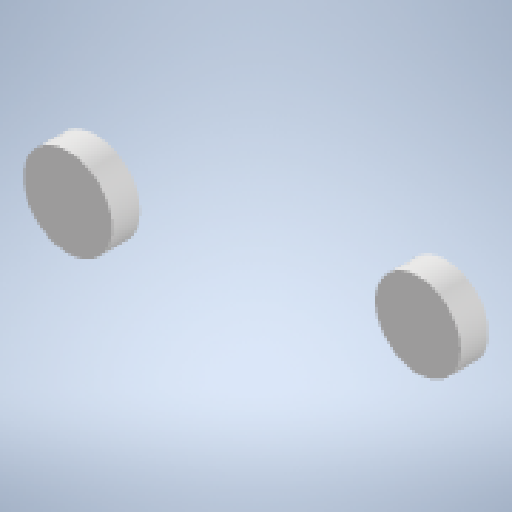
# Autodesk Inventor part: EyesGoma
Saved by Autodesk Inventor 2023 (Build 270158000, 158)
## iProperties
Created: 2022-11-10
Part Number: EyesGoma
Material: Generic
Document SubType Name: Modeling
Designer: reide
Density: 1 g/cm^3
Appearance: Default
Author: reide
Autodesk Inventor part; units mm, degrees
ref_plane "YZ Plane" through (0, 0, 0) normal (1, 0, 0) x (0, 1, 0)
ref_plane "XZ Plane" through (0, 0, 0) normal (0, 1, 0) x (-1, 0, 0)
ref_plane "XY Plane" through (0, 0, 0) normal (0, 0, 1) x (1, 0, 0)
sketch "Sketch1" plane through (0, 0, 0) normal (0, 0, 1) x (1, 0, 0)
  arc A0 (31.1669, -27.5722) -> (35.8875, -22.8773) centre (21.6106, -13.2427) ccw projected
  arc A1 (35.8875, -22.8773) -> (34.8455, -21.6033) centre (-10.0066, -59.351) ccw projected
  line L0 (31.177, -26.5722) -> (-3.0608, -26.5722) projected
  arc A2 (-3.0608, -26.5722) -> (-3.3209, -25.2629) centre (-5.1893, -26.3146) ccw projected
  arc A3 (-3.3209, -25.2629) -> (-1.1986, -22.6985) centre (-4.2539, -22.3302) ccw projected
  arc A4 (-1.1986, -22.6985) -> (27.6561, -16.2412) centre (3.0649, 25.9479) ccw projected
  arc A5 (34.8455, -21.6033) -> (38.4558, -17.1259) centre (14.65, -1.6245) ccw projected
  arc A6 (29.6868, -16.1644) -> (34.1879, -20.9364) centre (42.4009, -8.681) ccw projected
  arc A7 (29.6868, -16.1644) -> (32.1813, -14.508) centre (22.6557, -2.8691) ccw projected
  arc A8 (36.2837, -17.718) -> (32.1813, -14.508) centre (33.8318, -16.6251) ccw projected
  arc A9 (38.4558, -17.1259) -> (37.2045, -13.6874) centre (36.2505, -15.9815) ccw projected
  arc A10 (36.3385, -10.6874) -> (37.2045, -13.6874) centre (37.9725, -11.8408) ccw projected
  arc A11 (36.3385, -10.6874) -> (35.7081, 6.3323) centre (24.8683, -2.5908) ccw projected
  arc A12 (35.7081, 6.3323) -> (31.4684, 20.3428) centre (7.4536, 5.4291) ccw projected
  arc A13 (31.4684, 20.3428) -> (30.4027, 34.135) centre (0, 24.8485) ccw projected
  arc A14 (30.4027, 34.135) -> (17.0904, 32.0182) centre (26.8002, 13.8731) ccw projected
  arc A15 (17.0904, 32.0182) -> (-22.1361, 25.4066) centre (3.3472, -6.1143) ccw projected
  arc A16 (-22.1361, 25.4066) -> (-37.0956, 22.1531) centre (-24.1189, -1.495) ccw projected
  arc A17 (-37.0956, 22.1531) -> (-33.3027, 6.5823) centre (17.6972, 27.2528) ccw projected
  arc A18 (-33.3027, 6.5823) -> (-30.2964, -14.6197) centre (2.7199, 0.876) ccw projected
  arc A19 (-30.2964, -14.6197) -> (-18.2146, -23.7335) centre (-13.8358, -5.3636) ccw projected
  arc A20 (-18.2146, -23.7335) -> (-18.242, -27.5722) centre (-11.8923, -25.698) ccw projected
  line L1 (-44.3323, -27.5722) -> (-18.242, -27.5722) projected
  arc A21 (-44.3323, -27.5722) -> (-48.3323, -31.5722) centre (-44.3323, -31.5722) ccw projected
  line L2 (-48.3323, -136.5722) -> (-48.3323, -31.5722) projected
  arc A22 (-48.3323, -136.5722) -> (-44.3323, -140.5722) centre (-44.3323, -136.5722) ccw projected
  line L3 (92.8689, -140.5722) -> (-44.3323, -140.5722) projected
  line L4 (92.8689, -132.5706) -> (92.8689, -140.5722) projected
  line L5 (-38.9073, -132.5706) -> (92.8689, -132.5706) projected
  arc A23 (-40.9073, -130.5706) -> (-38.9073, -132.5706) centre (-38.9073, -130.5706) ccw projected
  line L6 (-40.9073, -37.5722) -> (-40.9073, -130.5706) projected
  arc A24 (-38.9073, -35.5722) -> (-40.9073, -37.5722) centre (-38.9073, -37.5722) ccw projected
  line L7 (92.8689, -35.5722) -> (-38.9073, -35.5722) projected
  line L8 (92.8689, -27.5722) -> (92.8689, -35.5722) projected
  line L9 (31.1669, -27.5722) -> (92.8689, -27.5722) projected
  arc A25 (10.4658, -0.0889) -> (9.3999, 0) centre (9.9366, 0) ccw projected
  arc A26 (10.4658, -0.0889) -> (10.6052, -0.4853) centre (11.0805, -0.0954) ccw projected
  arc A27 (10.6052, -0.4853) -> (12.2217, -0.0769) centre (11.2935, 0.1936) ccw projected
  arc A28 (14.0708, 0) -> (12.2217, -0.0769) centre (13.1642, -0.4715) ccw projected
  arc A29 (14.0708, 0) -> (15.5201, 0.876) centre (14.6273, 0.7161) ccw projected
  arc A30 (16.6059, 1.2358) -> (15.5201, 0.876) centre (16.0433, 1.1154) ccw projected
  arc A31 (13.0987, -0.702) -> (16.6059, 1.2358) centre (14.6781, 0.5822) ccw projected
  arc A32 (9.3999, 0) -> (13.0987, -0.702) centre (11.2957, -0.1065) ccw projected
  arc A33 (30.6396, 22.3597) -> (19.6168, 31.4004) centre (6.9952, 4.7714) ccw projected
  arc A34 (29.7697, 32.8548) -> (19.6168, 31.4004) centre (27.3183, 13.8041) ccw projected
  arc A35 (30.6396, 22.3597) -> (29.7697, 32.8548) centre (2.7, 25.3277) ccw projected
  line L10 (-7.4612, -26.5722) -> (-17.5392, -26.5722) projected
  arc A36 (-9.2038, -17.0917) -> (-15.8005, -20.192) centre (-6.8054, -30.7634) ccw projected
  arc A37 (-4.9865, -25.698) -> (-9.2038, -17.0917) centre (-21.6299, -28.5174) ccw projected
  arc A38 (-4.9865, -25.698) -> (-7.4612, -26.5722) centre (2.3833, -50.5016) ccw projected
  circle A39 centre (24.8683, 4.8774) radius 3.1762 projected
  circle A40 centre (0, 0) radius 3.3209 projected
  arc A41 (-23.3023, 23.7394) -> (-30.7067, 8.9093) centre (205.8131, -99.9189) ccw projected
  arc A42 (-35.2106, 21.0181) -> (-30.7067, 8.9093) centre (-10.6119, 23.2756) ccw projected
  arc A43 (-23.3023, 23.7394) -> (-35.2106, 21.0181) centre (-24.7545, 2.6784) ccw projected
  arc A44 (-3.7654, -23.5331) -> (-6.8054, -17.6334) centre (-5.1369, -20.5068) ccw projected
  arc A45 (-3.7654, -23.5331) -> (-6.8054, -17.6334) centre (-14.6416, -25.4043) ccw projected
  ellipse E0 centre (32.9155, 3.0366) end of major axis (36.6949, 3.0366) minor radius 3.3363 projected
  ellipse E1 centre (-8.3038, -4.7458) end of major axis (-4.0213, -3.7834) minor radius 3.3846 projected
  circle A46 centre (0, 0) radius 3.1549
  circle A47 centre (24.8683, 4.8774) radius 3.0174
  arc A48 (34.1879, -20.9364) -> (36.2837, -17.718) centre (26.5541, -13.6737) ccw projected
  arc A49 (27.6561, -16.2412) -> (33.9248, -23.5331) centre (40.7776, -11.3014) ccw projected
  arc A50 (31.177, -26.5722) -> (33.9248, -23.5331) centre (15.0767, -9.2529) ccw projected
  arc A51 (-15.8005, -20.192) -> (-17.5392, -26.5722) centre (-11.5031, -24.7901) ccw projected
  constraints: 2 centre point, 2 coincident
extrude "Extrusion1" add sketch "Sketch1" along normal blind 2 contours A46 | A47
body "Solid1"
